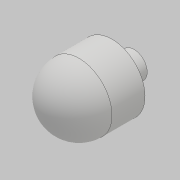
# Autodesk Inventor part: exercise2-7
Saved by Autodesk Inventor 2018 (Build 220112000, 112)
## iProperties
Created: 2020-09-21
Part Number: exercise2-7
Material: 一般
Document SubType Name: Modeling
Designer: 王鼎鈞
Density: 1 g/cm^3
Appearance: 預設
Author: 王鼎鈞
Autodesk Inventor part; units mm, degrees
ref_plane "YZ Plane" through (0, 0, 0) normal (1, 0, 0) x (0, 1, 0)
ref_plane "XZ Plane" through (0, 0, 0) normal (0, 1, 0) x (-1, 0, 0)
ref_plane "XY Plane" through (0, 0, 0) normal (0, 0, 1) x (1, 0, 0)
sketch "草圖1" plane through (0, 0, 0) normal (1, 0, 0) x (0, 1, 0)
  line L0 (0, -21.7279) -> (0, 3.6213) projected
  line L1 (-26.7279, 0) -> (33.6213, 0) projected
  line L2 (0, 0) -> (15, 0)
  line L3 (15, 0) -> (15, -15)
  line L4 (15, -15) -> (0, -15)
  line L5 (0, -15) -> (0, 0)
  line L6 (15, 0) -> (25, 0)
  line L7 (25, 0) -> (25, -6)
  line L8 (25, -6) -> (15, -6)
  line L9 (15, -6) -> (15, 0)
  arc A0 (-15, 0) -> (0, -15) centre (0, 0) ccw
  line L10 (-15, 0) -> (0, 0)
  dimension "d0" = 15
  dimension "d1" = 15
  dimension "d2" = 10
  dimension "d3" = 6
  constraints: 18 end point, 4 parallel, 3 horizontal, 2 perpendicular, 2 point on circle, 1 centre point, 1 coincident, 1 point on line
  measures "d0" distance of L3.end L4.end
  measures "d1" distance of L2.end L3.end
  measures "d2" distance of L7.end L8.end
  measures "d3" distance of L6.end L7.end
revolve "迴轉1" add sketch "草圖1" angle 360 about axis through (0, 0, 0) along (0, 1, 0)
